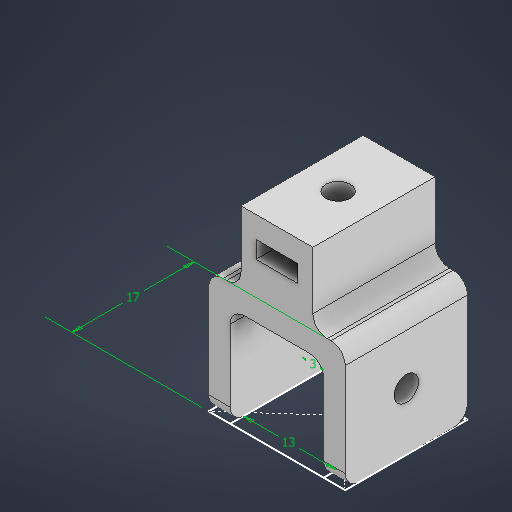
# Autodesk Inventor part: Idlert Tensioner
Saved by Autodesk Inventor 2025.1 (Build 291241000, 241)
## iProperties
Created: 2025-01-23
Part Number: Idlert Tensioner
Material: Generic
Document SubType Name: Modeling
Designer: jerem
Density: 1 g/cm^3
Appearance: Default
Author: jerem
## iProperties of the stored document Idlert Tensioner_3DPrint.ipt
Created: 2025-01-23
Part Number: Idlert Tensioner_3DPrint
Material: Generic
Document SubType Name: Modeling
Designer: jerem
Density: 1 g/cm^3
Appearance: Default
Author: jerem
Autodesk Inventor part; units mm, degrees
ref_plane "YZ Plane" through (0, 0, 0) normal (1, 0, 0) x (0, 1, 0)
ref_plane "XZ Plane" through (0, 0, 0) normal (0, 1, 0) x (-1, 0, 0)
ref_plane "XY Plane" through (0, 0, 0) normal (0, 0, 1) x (1, 0, 0)
sketch "Sketch3" plane through (0, 0, 0) normal (0, 1, 0) x (-1, 0, 0)
  line L0 (-9.5, 8.5) -> (9.5, 8.5)
  line L1 (9.5, 8.5) -> (9.5, -8.5)
  line L2 (9.5, -8.5) -> (-9.5, -8.5)
  line L3 (-9.5, -8.5) -> (-9.5, 8.5)
  line L4 (-9.5, 8.5) -> (9.5, -8.5) construction
  line L5 (9.5, 8.5) -> (-9.5, -8.5) construction
  line L6 (6.5, -8.5) -> (6.5, 8.5)
  line L7 (-6.5, 8.5) -> (-6.5, -8.5)
  line L8 (-6.5, -5.8158) -> (6.5, -5.8158) construction
  point P0 (0, 0)
  dimension "d12" = 17
  dimension "d17" = 3
  dimension "d36" = 13
  constraints: 18 end point, 8 point on line, 3 perpendicular, 2 horizontal, 2 midpoint, 2 parallel
  measures "d12" distance of L0.end L1.end
  measures "d17" distance between parallel lines of L1 L6
  measures "d36" distance between parallel lines of L7 L6
extrude "Extrusion3" add sketch "Sketch3" along normal blind 17
sketch "Sketch4" plane through (9.5, 0, 8.5) normal (1, 0, 0) x (0, 0, -1)
  line L0 (8.5, 0) -> (8.5, 8) construction
  circle A0 centre (8.5, 8) radius 1.7
  line L1 (0, 0) -> (17, 0) projected
  dimension "d15" = 3.4
  dimension "d16" = 8
  constraints: 2 end point, 1 centre point, 1 coincident, 1 vertical
  measures "d15" diameter of A0
  measures "d16" distance from line of L1 L0.end
extrude "Extrusion4" cut sketch "Sketch3" along normal blind 14 contours L0 L6 L2 L7
extrude "Extrusion5" cut sketch "Sketch4" against normal through all
sketch "Sketch5" plane through (0, 17, 0) normal (0, 1, 0) x (1, 0, 0)
  line L0 (-6.5, -8.5) -> (6.5, -8.5) projected
  line L1 (-5, 8.5) -> (5, 8.5)
  line L2 (5, 8.5) -> (5, -8.5)
  line L3 (5, -8.5) -> (-5, -8.5)
  line L4 (-5, -8.5) -> (-5, 8.5)
  line L5 (-5, 8.5) -> (5, -8.5) construction
  line L6 (5, 8.5) -> (-5, -8.5) construction
  point P0 (0, 0)
  dimension "d22" = 10
  constraints: 12 end point, 2 midpoint, 2 parallel, 1 horizontal, 1 perpendicular, 1 point on line
  measures "d22" distance of L2.end L3.end
extrude "Extrusion6" add sketch "Sketch5" along normal blind 10
sketch "Sketch6" plane through (9.5, 0, 8.5) normal (0, 0, 1) x (1, 0, 0)
  line L0 (-6.6, 24) -> (-12.4, 24)
  line L1 (-12.4, 24) -> (-12.4, 21.6)
  line L2 (-12.4, 21.6) -> (-6.6, 21.6)
  line L3 (-6.6, 21.6) -> (-6.6, 24)
  line L4 (-6.6, 24) -> (-12.4, 21.6) construction
  line L5 (-12.4, 24) -> (-6.6, 21.6) construction
  line L6 (-9.5, 24) -> (-9.5, 27) construction
  line L7 (-4.5, 27) -> (-14.5, 27) construction
  line L8 (-19, 17) -> (-14.5, 17) construction
  point P0 (-9.5, 0)
  point P1 (-9.5, 22.8)
  dimension "d25" = 5.8
  dimension "d26" = 2.4
  dimension "d34" = 3
  constraints: 14 end point, 4 midpoint, 2 parallel, 2 perpendicular, 1 horizontal
  measures "d25" distance of L2.end L1.end
  measures "d26" distance of L1.end L0.end
  measures "d34" distance between parallel lines of L7 L0
extrude "Extrusion7" cut sketch "Sketch6" against normal blind 11.3
sketch "Sketch7" plane through (0, 27, 0) normal (0, 1, 0) x (1, 0, 0)
  circle A0 centre (0, 0) radius 1.7
  dimension "d30" = 3.4
  constraints: 1 centre point, 1 coincident
  measures "d30" diameter of A0
extrude "Extrusion8" cut sketch "Sketch7" against normal through all
fillet "Fillet1" radius 2 6 edges at (5, 17, 0) (-5, 17, 0) (-9.5, 17, 0) (-6.5, 14, 0) (9.5, 17, 0) (6.5, 14, 0)
fillet "Fillet2" radius 2 4 edges at (-8, 0, -8.5) (8, 0, -8.5) (-8, 0, 8.5) (8, 0, 8.5)
body "Solid2"
